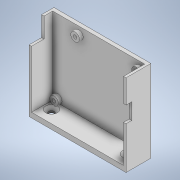
# Autodesk Inventor part: Electronicsmount
Saved by Autodesk Inventor 2021 (Build 250183000, 183)
## iProperties
Created: 2024-06-30
Part Number: Electronicsmount
Material: Generic
Document SubType Name: Modeling
Designer: Lukas
Density: 1 g/cm^3
Appearance: Default
Author: Lukas
Autodesk Inventor part; units mm, degrees
ref_plane "YZ Plane" through (0, 0, 0) normal (1, 0, 0) x (0, 1, 0)
ref_plane "XZ Plane" through (0, 0, 0) normal (0, 1, 0) x (-1, 0, 0)
ref_plane "XY Plane" through (0, 0, 0) normal (0, 0, 1) x (1, 0, 0)
sketch "Sketch1" plane through (0, 0, 0) normal (0, 0, 1) x (1, 0, 0)
  line L0 (-39, 33) -> (39, 33)
  line L1 (39, 33) -> (39, -33)
  line L2 (39, -33) -> (-39, -33)
  line L3 (-39, -33) -> (-39, 33)
  point P0 (0, 0)
  point P1 (0, 33)
  point P2 (-39, 0)
  dimension "d0" = 78
  dimension "d1" = 66
  constraints: 8 end point, 2 midpoint, 2 parallel, 1 horizontal, 1 horizontal alignment, 1 perpendicular, 1 vertical alignment
  measures "d0" distance of L0.start L0.end
  measures "d1" distance of L0.end L1.end
extrude "Extrusion1" add sketch "Sketch1" along normal blind 3
sketch "Sketch2" plane through (0, 0, 3) normal (0, 0, 1) x (1, 0, 0)
  line L0 (-39, -33) -> (39, -33) projected
  line L1 (-39, -33) -> (39, -33)
  line L2 (39, -33) -> (39, -29)
  line L3 (39, -29) -> (-39, -29)
  line L4 (-39, -29) -> (-39, -33)
  line L5 (39, -33) -> (39, 33) projected
  circle A0 centre (-16, 27) radius 3.5
  circle A1 centre (-33, -26) radius 3.5
  circle A2 centre (33, -26) radius 3.5
  circle A3 centre (33, 27) radius 3.5
  circle A4 centre (33, 27) radius 1.4
  circle A5 centre (33, -26) radius 1.4
  circle A6 centre (-33, -26) radius 1.4
  circle A7 centre (-16, 27) radius 1.4
  line L6 (-39, 33) -> (-39, -33) projected
  line L7 (39, 33) -> (-39, 33) projected
  line L8 (37, -29) -> (37, 33)
  line L9 (-37, -29) -> (-37, 33)
  point P0 (0, 0)
  dimension "d4" = 4
  dimension "d5" = 49
  dimension "d6" = 66
  dimension "d7" = 53
  dimension "d8" = 6
  dimension "d9" = 6
  dimension "d11" = 2.8
  dimension "d12" = 7
  dimension "d22" = 2
  dimension "d23" = 2
  dimension "d27" = 3
  constraints: 12 end point, 8 centre point, 6 equal radius, 5 point on line, 4 coincident, 3 perpendicular, 2 horizontal alignment, 2 parallel, 1 horizontal, 1 vertical alignment
  measures "d4" distance of L1.end L2.end
  measures "d5" distance of A3.centre A0.centre
  measures "d6" distance of A2.centre A1.centre
  measures "d7" distance of A3.centre A2.centre
  measures "d8" distance from line of L5 A3.centre
  measures "d9" distance from line of L6 A1.centre
  measures "d11" diameter of A6
  measures "d12" diameter of A1
  measures "d22" distance between parallel lines of L5 L8
  measures "d23" distance between parallel lines of L6 L9
  measures "d27" distance from line of A2.centre L3
extrude "Extrusion2" add sketch "Sketch2" along normal blind 3 contours A1 L3 | L3 A1 | A2 L3 | L3 A2 | A0 | A3
extrude "Extrusion3" add sketch "Sketch2" along normal blind 17 contours L4 L3 A1 A2 L2 L0 | L6 L7 L9 L3 | L3 L8 L7 L5 | L3 A1 | A2 L3 picked at (-33.3722, -29.1057) picked at (32.6278, -29.1057)
sketch "Sketch3" plane through (-39, -33, 0) normal (0, -1, 0) x (1, 0, 0)
  circle A0 centre (8, 10) radius 2.25
  circle A1 centre (70, 10) radius 2.25
  line L0 (0, 0) -> (0, 20) projected
  line L1 (78, 0) -> (78, 20) projected
  point P0 (39, 0)
  point P1 (0, 10)
  dimension "d17" = 8
  dimension "d18" = 8
  dimension "d19" = 4.5
  constraints: 2 centre point, 2 horizontal alignment, 1 equal radius, 1 midpoint
  measures "d17" distance from line of L0 A0.centre
  measures "d18" distance from line of L1 A1.centre
  measures "d19" diameter of A1
extrude "Extrusion4" cut sketch "Sketch3" against normal through all
chamfer "Chamfer1" distance 2.5 angle 45 2 edges at (-33.25, -29, 10) (28.75, -29, 10)
sketch "Sketch4" plane through (39, -33, 0) normal (-1, 0, 0) x (0, 0, 1)
  line L0 (20, 47) -> (15.4, 47)
  line L1 (15.4, 47) -> (15.4, 34)
  line L2 (15.4, 34) -> (20, 34)
  line L3 (20, 34) -> (20, 47)
  line L4 (20, 66) -> (20, 0) projected
  line L5 (6, 8.4) -> (6, 5.6) projected
  line L6 (3, 5.6) -> (3, 8.4) projected
  line L7 (6, 61.4) -> (6, 58.6) projected
  line L8 (3, 58.6) -> (3, 61.4) projected
  point P0 (0, 33)
  point P1 (6, 7)
  point P2 (6, 60)
  dimension "d29" = 13
  dimension "d30" = 9.4
  dimension "d37" = 13
  constraints: 8 end point, 2 midpoint, 2 parallel, 1 horizontal, 1 perpendicular, 1 point on line
  measures "d29" distance of L0.end L1.end
  measures "d30" distance between parallel lines of L5 L1
  measures "d37" distance from line of point (6, 60) L0
extrude "Extrusion5" cut sketch "Sketch4" along normal up to surface (76 mm away)
sketch "Sketch5" plane through (-39, -33, 0) normal (1, 0, 0) x (0, 0, -1)
  line L0 (0, 66) -> (-20, 66) projected
  line L1 (-20, 66) -> (-10, 66)
  line L2 (-10, 66) -> (-10, 50)
  line L3 (-10, 50) -> (-20, 50)
  line L4 (-20, 50) -> (-20, 66)
  line L5 (-6, 58.6) -> (-6, 61.4) projected
  line L6 (-3, 61.4) -> (-3, 58.6) projected
  point P0 (0, 33)
  point P1 (-6, 60)
  dimension "d33" = 10
  dimension "d34" = 4
  constraints: 8 end point, 2 parallel, 1 horizontal, 1 midpoint, 1 perpendicular
  measures "d33" distance from line of L3 point (-6, 60)
  measures "d34" distance between parallel lines of L5 L2
extrude "Extrusion6" cut sketch "Sketch5" along normal up to surface (76 mm away)
equation "\"d8\" = d9"
equation "\"d23\" = d22"
equation "\"d18\" = d17"
body "Solid1"
